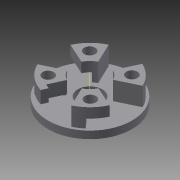
# Autodesk Inventor part: new male 4 bay con
Saved by Autodesk Inventor 2015 (Build 190159000, 159)
## iProperties
Created: 2014-11-16
Part Number: new male 4 bay con
Material: Generic
Document SubType Name: Modeling
Designer: ericd_000
Density: 1 g/cm^3
Appearance: Default
Author: ericd_000
Autodesk Inventor part; units mm, degrees
ref_plane "YZ Plane" through (0, 0, 0) normal (1, 0, 0) x (0, 1, 0)
ref_plane "XZ Plane" through (0, 0, 0) normal (0, 1, 0) x (-1, 0, 0)
ref_plane "XY Plane" through (0, 0, 0) normal (0, 0, 1) x (1, 0, 0)
sketch "Sketch1" plane through (0, 0, 0) normal (0, 0, 1) x (1, 0, 0)
  circle A0 centre (0, 0) radius 34
  dimension "d0" = 68
  constraints: 1 centre point, 1 coincident
  measures "d0" diameter of A0
extrude "Extrusion1" add sketch "Sketch1" along normal blind 6
sketch "Sketch2" plane through (0, 0, 6) normal (0, 0, 1) x (1, 0, 0)
  circle A0 centre (0, 0) radius 34
  circle A1 centre (0, 0) radius 34 projected
  line L0 (0, 0) -> (30.6997, 14.6126) construction
  line L1 (0, 0) -> (25.8716, 22.0604) construction
  line L2 (25.8716, 22.0604) -> (10.653, 9.0837)
  line L3 (30.6997, 14.6126) -> (12.641, 6.017)
  arc A2 (30.6997, 14.6126) -> (25.8716, 22.0604) centre (0, 0) ccw
  arc A3 (12.641, 6.017) -> (10.653, 9.0837) centre (0, 0) ccw
  dimension "d3" = 15
  dimension "d4" = 20
  constraints: 8 end point, 8 point on circle, 3 centre point, 3 concentric, 2 point on line, 1 coincident
  measures "d3" angle of L0 L1
  measures "d4" distance of L1.end L2.end
extrude "Extrusion2" add sketch "Sketch2" along normal blind 15 contours L3 A3 L2 A0 picked at (22.8031, 15.025)
sketch "Sketch3" plane through (10.653, 9.0837, 21) normal (-0.6488347, 0.7609293, 0) x (0.7609293, 0.6488347, 0)
  line L0 (0, 15) -> (0, 0) projected
  line L1 (20, 0) -> (0, 0)
  line L2 (0, 0) -> (0, 8)
  line L3 (0, 8) -> (20, 8)
  line L4 (20, 8) -> (20, 0)
  line L5 (-14, 25.2) -> (-14, -4.2) projected
  line L6 (-48, 15) -> (20, 15) projected
  point P0 (-14, 21)
  point P1 (18.8415, 15)
  dimension "d7" = 8
  dimension "d26" = 7
  constraints: 8 end point, 2 parallel, 1 horizontal, 1 perpendicular, 1 point on line
  measures "d7" distance between parallel lines of L3 L1
  measures "d26" distance between parallel lines of L6 L3
revolve "Revolution1" add sketch "Sketch3" angle 25 about axis through (0, 0, 6) along (0, 0, 1)
sketch "Sketch4" plane through (0, 0, 21) normal (0, 0, 1) x (1, 0, 0)
  circle A0 centre (16.8356, 17.1044) radius 4.5
  arc A1 (12.641, 6.017) -> (5.816, 12.7348) centre (0, 0) ccw projected
  arc A2 (30.6997, 14.6126) -> (14.1245, 30.9273) centre (0, 0) ccw projected
  line L0 (12.641, 6.017) -> (30.6997, 14.6126) projected
  line L1 (5.816, 12.7348) -> (14.1245, 30.9273) projected
  arc A3 (21.6704, 10.3148) -> (9.9702, 21.831) centre (0, 0) ccw construction
  circle A4 centre (0, 0) radius 34 construction
  line L2 (23.8505, 24.2313) -> (19.6046, 19.9177) construction
  dimension "d12" = 9
  constraints: 5 point on circle, 2 centre point, 2 end point, 2 midpoint, 1 concentric, 1 line through centre, 1 point on line
  measures "d12" diameter of A0
extrude "Extrusion3" cut sketch "Sketch4" against normal blind 12 contours A0
pattern_circular "Circular Pattern2" count 4 over 360 about axis through (0, 0, 6) along (0, 0, 1) of "Revolution1", "Extrusion3", "Extrusion2"
sketch "Sketch5" plane through (0, 0, 0) normal (0, 0, -1) x (-1, 0, 0)
  circle A0 centre (0, 0) radius 10
  dimension "d23" = 20
  constraints: 1 centre point, 1 coincident
  measures "d23" diameter of A0
extrude "Extrusion4" cut sketch "Sketch5" against normal blind 10
sketch "Sketch6" plane through (-14.1245, -30.9273, 13) normal (0, 0, -1) x (-0.9096266, 0.4154268, 0)
  line L0 (11.7881, 8.7204) -> (14.369, 3.1855) projected
  line L1 (0, 0) -> (0, 20)
  arc A0 (0, 0) -> (14.369, 3.1855) centre (0, 34) ccw
  arc A1 (0, 20) -> (5.9167, 21.3117) centre (0, 34) ccw projected
  arc A2 (0, 20) -> (5.9167, 21.3117) centre (0, 34) ccw
  arc A3 (0, 0) -> (14.369, 3.1855) centre (0, 34) ccw projected
  arc A4 (8.4204, 15.9424) -> (11.7881, 8.7204) centre (8.2085, 11.4474) ccw
  arc A5 (8.4204, 15.9424) -> (11.7881, 8.7204) centre (8.2085, 11.4474) ccw projected
  line L2 (14.369, 3.1855) -> (11.7881, 8.7204)
  line L3 (8.4204, 15.9424) -> (5.9167, 21.3117)
  point P0 (0, 34)
  constraints: 9 point on circle, 6 end point, 4 concentric, 3 centre point, 2 collinear, 1 vertical
extrude "Extrusion5" add sketch "Sketch6" along normal blind 2
sketch "Sketch7" plane through (0, 0, 21) normal (0, 0, 1) x (0.7126851, -0.7014841, 0)
  line L0 (11.6287, -31.9495) -> (9.1517, -25.1441)
  line L1 (4.7883, -13.1557) -> (11.6287, -31.9495) projected
  line L2 (12.9105, -23.776) -> (15.3067, -30.3596)
  arc A0 (11.6287, -31.9495) -> (15.3067, -30.3596) centre (0, 0) ccw
  line L3 (12.9105, -23.776) -> (9.1517, -25.1441)
  arc A1 (-11.6287, -31.9495) -> (11.6287, -31.9495) centre (0, 0) ccw projected
  dimension "d29" = 4
  constraints: 6 end point, 2 perpendicular, 2 point on circle, 1 centre point, 1 concentric, 1 point on line
  measures "d29" distance of L2.start L0.end
extrude "Extrusion6" add sketch "Sketch7" against normal blind 10
sketch "Sketch8" plane through (-30.6997, -14.6126, 21) normal (0, 0, 1) x (0.9029321, 0.4297832, 0)
  circle A0 centre (34, 0) radius 34 projected
  circle A1 centre (34, 0) radius 34
  circle A2 centre (34, 0) radius 10 projected
  circle A3 centre (34, 0) radius 32
  dimension "d32" = 2
  constraints: 2 centre point, 2 coincident, 1 concentric
  measures "d32" radial gap between concentric circles of A0 A3
extrude "Extrusion7" cut sketch "Sketch8" against normal up to surface (15 mm away) contours A0
body "Solid1"
